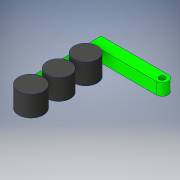
# Autodesk Inventor part: arm
Saved by Autodesk Inventor 2016 (Build 200138000, 138)
## iProperties
Created: 2018-01-12
Part Number: arm
Material: Aluminum 6061
Document SubType Name: Modeling
Designer: New User
Density: 2.7 g/cm^3
Appearance: Aluminum - Flat
Mass: 1109.3 g
Surface Area: 532.958 cm^2
Volume: 410.85 cm^3
Author: New User
Autodesk Inventor part; units mm, degrees
ref_plane "YZ Plane" through (0, 0, 0) normal (1, 0, 0) x (0, 1, 0)
ref_plane "XZ Plane" through (0, 0, 0) normal (0, 1, 0) x (-1, 0, 0)
ref_plane "XY Plane" through (0, 0, 0) normal (0, 0, 1) x (1, 0, 0)
sketch "Sketch1" plane through (0, 0, 0) normal (0, 1, 0) x (-1, 0, 0)
  line L0 (0, 0) -> (-25.4, 0)
  line L1 (-25.4, 0) -> (-25.4, -152.4)
  line L2 (-25.4, -152.4) -> (-157.48, -152.4)
  line L3 (-157.48, -152.4) -> (-157.48, -177.8)
  line L4 (-157.48, -177.8) -> (0, -177.8)
  line L5 (0, -177.8) -> (0, 0)
  dimension "d0" = 152.4
  dimension "d1" = 132.08
  dimension "d2" = 25.4
  constraints: 12 end point, 6 perpendicular, 1 horizontal
  measures "d0" distance of L0.end L1.end
  measures "d1" distance of L1.end L2.end
  measures "d2" distance of L2.end L3.end
extrude "Extrusion1" add sketch "Sketch1" along normal blind 25.4
sketch "Sketch2" plane through (0, 25.4, 0) normal (0, 1, 0) x (1, 0, 0)
  circle A0 centre (144.78, 165.1) radius 6.35
  line L0 (157.48, 152.4) -> (157.48, 177.8) projected
  line L1 (157.48, 177.8) -> (0, 177.8) projected
  point P0 (0, 0)
  dimension "d5" = 12.7
  dimension "d6" = 12.7
  dimension "d7" = 12.7
  constraints: 1 centre point
  measures "d5" diameter of A0
  measures "d6" distance from line of L0 A0.centre
  measures "d7" distance from line of L1 A0.centre
extrude "Extrusion2" cut sketch "Sketch2" against normal blind 39.6875
fillet "Fillet1" radius 12.7 2 edges at (157.48, 12.7, -152.4) (157.48, 12.7, -177.8)
sketch "Sketch3" plane through (0, 25.4, 0) normal (0, 1, 0) x (1, 0, 0)
  line L0 (0, 0) -> (25.4, 0) projected
  circle A0 centre (25.4, 0) radius 26.9542
  circle A1 centre (25.4, 60.256) radius 25.4
  line L1 (25.4, 0) -> (25.4, 152.4) projected
  circle A2 centre (25.4, 118.6489) radius 25.4
  dimension "d11" = 50.8
  constraints: 3 centre point, 1 equal radius, 1 point on line
  measures "d11" diameter of A2
extrude "Extrusion3" add sketch "Sketch3" along normal blind 11.1125 and the other way blind 33.3375
body "Solid1"
